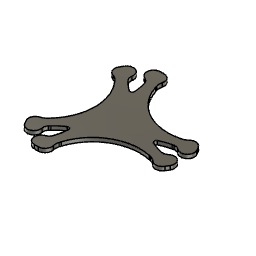
slot_solve (Autodesk Fusion 360 design; units mm, degrees)
Autodesk Fusion 360 part; units mm, degrees
sketch "Sketch1" plane through (0, 0, 0) normal (0, 0, 1) x (1, 0, 0)
  line L0 (0, 0) -> (24.4074, 5.411) construction
  line L1 (1.75, 0) -> (22.5, 0) construction
  dimension "d1" = 25
  dimension "d2" = 12.5
  constraint coincident L0.start origin
  measures "d1" distance of L0.start L0.end
  measures "d2" angle of L0 L1
ref_plane "WorkPlane1" through (0, 0, 20) normal (0, 0, 1) x (1, 0, 0)
sketch "Sketch2" plane through (0, 0, 20) normal (0, 0, 1) x (1, 0, 0)
  line L0 (0, 0) -> (16.8898, 18.4319) construction
  line L1 (1.75, 0) -> (22.5, 0) construction
  dimension "d4" = 25
  dimension "d5" = 47.5
  constraint coincident L0.start origin
  measures "d4" distance of L0.start L0.end
  measures "d5" angle of L0 L1
sketch "Sketch3" plane through (0, 0, 0) normal (0, 0, 1) x (1, 0, 0)
  line L0 (24.4074, 5.411, 0) -> (16.8898, 18.4319, 20) construction
  point P0 (24.4074, 5.411)
  point P1 (16.8898, 18.4319)
ref_plane "WorkPlane2" through (24.4074, 5.411, 0) normal (-0.300451, 0.520397, 0.799322) x (-0.866025, -0.5, 0)
sketch "Sketch4" plane through (24.4074, 5.411, 0) normal (-0.300451, 0.520397, 0.799322) x (-0.866025, -0.5, 0)
  circle A0 centre (0, 0) radius 0.9
  dimension "d7" = 1.8
  constraint coincident A0.centre origin
  measures "d7" diameter of A0
extrude "Extrude1" add sketch "Sketch4" along normal mid plane 20 makes body 1
ref_plane "WorkPlane3" through (0, 0, -1.6) normal (0, 0, 1) x (1, 0, 0)
sketch "Sketch6" plane through (0, 0, -1.6) normal (0, 0, 1) x (1, 0, 0)
  ellipse E0 centre (25.0088, 4.3693) end of major axis (25.5718, 3.3942) minor radius 0.9
sketch "Sketch5" plane through (0, 0, 0) normal (0, 0, 1) x (1, 0, 0)
  ellipse E0 centre (24.4074, 5.411) end of major axis (24.9704, 4.4359) minor radius 0.9
  line L0 (23.515, 5.1567) -> (24.3424, 3.7236) construction
  arc A0 (24.3424, 3.7236) -> (25.9012, 4.6236) centre (25.1218, 4.1736) ccw construction
  line L1 (25.9012, 4.6236) -> (25.0738, 6.0567) construction
  arc A1 (25.0738, 6.0567) -> (23.515, 5.1567) centre (24.2944, 5.6067) ccw construction
  line L2 (24.2944, 5.6067) -> (25.1218, 4.1736) construction
  ellipse E1 centre (25.0088, 4.3693) end of major axis (25.5718, 3.3942) minor radius 0.9
  line L3 (0, 0) -> (24.4074, 5.411) construction
  line L4 (24.7081, 4.8902) -> (0, 0) construction
  line L5 (24.4074, 5.411) -> (24.5179, 4.8525) construction
  line L6 (14.0336, 5.0778) -> (14.8647, 1.3288) construction
  line L7 (14.8647, 1.3288) -> (22.6751, 3.0603) construction
  line L8 (22.6751, 3.0603) -> (21.844, 6.8093) construction
  line L9 (21.844, 6.8093) -> (14.0336, 5.0778) construction
  line L10 (20.3215, 2.4566) -> (21.0327, 2.6143)
  arc A2 (23.1558, 2.0418) -> (27.6333, 5.6236) centre (25.1218, 4.1736) ccw
  line L11 (27.6333, 5.6236) -> (26.8059, 7.0567)
  line L12 (22.6103, 2.7236) -> (22.6103, 2.7236)
  line L13 (20.167, 6.5195) -> (19.4558, 6.3618)
  arc A3 (20.167, 6.5195) -> (22.2452, 7.6587) centre (19.2493, 10.6588) ccw
  arc A4 (23.1558, 2.0418) -> (21.0327, 2.6143) centre (21.5465, 0.2968) ccw
  arc A5 (26.8059, 7.0567) -> (22.2452, 7.6587) centre (24.2944, 5.6067) ccw
  circle A6 centre (15.612, 5.4892) radius 0.4 construction
  line L14 (1.75, 0) -> (22.5, 0)
  line L15 (20.3215, -2.4566) -> (21.0327, -2.6143)
  arc A7 (21.0327, -2.6143) -> (23.1558, -2.0418) centre (21.5465, -0.2968) ccw
  arc A8 (27.6333, -5.6236) -> (23.1558, -2.0418) centre (25.1218, -4.1736) ccw
  line L16 (27.6333, -5.6236) -> (26.8059, -7.0567)
  arc A9 (22.2452, -7.6587) -> (26.8059, -7.0567) centre (24.2944, -5.6067) ccw
  arc A10 (22.2452, -7.6587) -> (20.167, -6.5195) centre (19.2493, -10.6588) ccw
  line L17 (20.167, -6.5195) -> (19.4558, -6.3618)
  arc A11 (-4.2184, 20.0301) -> (19.4558, 6.3618) centre (15.0768, 26.1138) ccw
  arc A12 (20.3215, 2.4566) -> (15.6882, 0.818) centre (24.7004, -17.2954) ccw
  arc A13 (15.6882, 0.818) -> (15.6882, -0.818) centre (16.0952, 0) ccw
  arc A14 (15.6882, -0.818) -> (20.3215, -2.4566) centre (24.7004, 17.2954) ccw
  line L18 (-4.4375, 20.7248) -> (-4.2184, 20.0301)
  arc A15 (-4.49, 23.0943) -> (-4.4375, 20.7248) centre (-0.3938, 21.9998) ccw
  arc A16 (-4.49, 23.0943) -> (-7.2917, 26.7429) centre (-7.2917, 23.8429) ccw
  line L19 (-8.9464, 26.7429) -> (-7.2917, 26.7429)
  arc A17 (-8.9464, 26.7429) -> (-9.8096, 21.0744) centre (-8.9464, 23.8429) ccw
  arc A18 (-8.2523, 19.522) -> (-9.8096, 21.0744) centre (-10.5162, 18.8082) ccw
  line L20 (-8.0333, 18.8273) -> (-8.2523, 19.522)
  arc A19 (-7.1357, 13.9954) -> (-8.0333, 18.8273) centre (-27.3285, 12.7435) ccw
  arc A20 (-8.5526, 13.1774) -> (-7.1357, 13.9954) centre (-8.0476, 13.9389) ccw
  arc A21 (-12.2882, 16.3706) -> (-8.5526, 13.1774) centre (2.6281, 30.0389) ccw
  line L21 (-12.2882, 16.3706) -> (-12.7804, 16.9077)
  arc A22 (-13.3461, 19.0326) -> (-12.7804, 16.9077) centre (-11.0303, 18.5114) ccw
  arc A23 (-13.3461, 19.0326) -> (-18.6868, 21.1193) centre (-16.1754, 19.6693) ccw
  line L22 (-18.6868, 21.1193) -> (-19.5142, 19.6863)
  arc A24 (-19.5142, 19.6863) -> (-17.7553, 15.4356) centre (-17.0027, 18.2363) ccw
  arc A25 (-15.7295, 14.2054) -> (-17.7553, 15.4356) centre (-18.8555, 11.341) ccw
  line L23 (-15.7295, 14.2054) -> (-15.2374, 13.6683)
  arc A26 (-15.2374, -13.6683) -> (-15.2374, 13.6683) centre (-30.1537, 0) ccw
  line L24 (-15.7295, -14.2054) -> (-15.2374, -13.6683)
  arc A27 (-17.7553, -15.4356) -> (-15.7295, -14.2054) centre (-18.8555, -11.341) ccw
  arc A28 (-17.7553, -15.4356) -> (-19.5142, -19.6863) centre (-17.0027, -18.2363) ccw
  line L25 (-18.6868, -21.1193) -> (-19.5142, -19.6863)
  arc A29 (-18.6868, -21.1193) -> (-13.3461, -19.0326) centre (-16.1754, -19.6693) ccw
  arc A30 (-12.7804, -16.9077) -> (-13.3461, -19.0326) centre (-11.0303, -18.5114) ccw
  line L26 (-12.2882, -16.3706) -> (-12.7804, -16.9077)
  arc A31 (-8.5526, -13.1774) -> (-12.2882, -16.3706) centre (2.6281, -30.0389) ccw
  arc A32 (-7.1357, -13.9954) -> (-8.5526, -13.1774) centre (-8.0476, -13.9389) ccw
  arc A33 (-8.0333, -18.8273) -> (-7.1357, -13.9954) centre (-27.3285, -12.7435) ccw
  line L27 (-8.0333, -18.8273) -> (-8.2523, -19.522)
  arc A34 (-9.8096, -21.0744) -> (-8.2523, -19.522) centre (-10.5162, -18.8082) ccw
  arc A35 (-9.8096, -21.0744) -> (-8.9464, -26.7429) centre (-8.9464, -23.8429) ccw
  line L28 (-8.9464, -26.7429) -> (-7.2917, -26.7429)
  arc A36 (-7.2917, -26.7429) -> (-4.49, -23.0943) centre (-7.2917, -23.8429) ccw
  arc A37 (-4.4375, -20.7248) -> (-4.49, -23.0943) centre (-0.3938, -21.9998) ccw
  line L29 (-4.4375, -20.7248) -> (-4.2184, -20.0301)
  arc A38 (19.4558, -6.3618) -> (-4.2184, -20.0301) centre (15.0768, -26.1138) ccw
  point P0 (24.7081, 4.8902)
  point P1 (14.4492, 3.2033)
  dimension "d11" = 107.5
  dimension "d12" = 0.1939
  dimension "d13" = 0.5693
  dimension "d14" = 3.84
  dimension "d15" = 8
  dimension "d16" = 14.8
  dimension "d17" = 2
  dimension "d19" = 1.7
  dimension "d21" = 1.7
  dimension "d22" = 2
  dimension "d23" = 2
  dimension "d24" = 1.63
  dimension "d25" = 0.06
  dimension "d26" = 0.8
  dimension "d38" = 360
  constraint tangent L0 A0
  constraint tangent A0 L1
  constraint parallel L0 L1
  constraint tangent L1 A1
  constraint tangent L0 A1
  constraint tangent E0 L1
  constraint tangent L1 E1
  constraint tangent E0 L0
  constraint tangent E0 A1
  constraint tangent A0 E1
  constraint coincident L2 P0
  constraint midpoint L2 P0
  constraint coincident P0 L4.start
  constraint coincident L3.start L4.end
  constraint coincident E0.centre L3.end
  constraint coincident L4 L5.end
  constraint perpendicular L4 L5
  constraint perpendicular L6 L7
  constraint parallel L6 L8
  constraint parallel L7 L9
  constraint parallel L3 L9
  constraint midpoint L6 P1
  constraint coincident L3 P1
  constraint parallel L7 L10
  constraint parallel L9 L13
  constraint tangent L13 A3
  constraint tangent A3 A5
  constraint tangent L10 A4
  constraint tangent A2 A4
  constraint concentric A0 A2
  constraint parallel L1 L11
  constraint concentric A1 A5
  constraint parallel L0 L12
  constraint tangent L11 A5
  constraint tangent A2 L11
  constraint symmetric L10.start L14 L15.start
  constraint symmetric L10.end L14 L15.end
  constraint symmetric A2.end L14 A8.start
  constraint symmetric A2 L14 A8
  constraint symmetric L11.end L14 L16.end
  constraint symmetric L13.start L14 A10.end
  constraint symmetric L13.end L14 L17.end
  constraint symmetric A3.end L14 A9.start
  constraint symmetric A3 L14 A10
  constraint symmetric A2.start L14 A7.end
  constraint symmetric A4 L14 A7
  constraint symmetric A5 L14 A9
  constraint tangent L13 A11
  constraint tangent A6 A11
  constraint equal L10 L13
  constraint tangent L10 A12
  constraint equal A11 A12
  constraint tangent A12 A13
  constraint symmetric L14 A12.end A13.end
  constraint symmetric L14 A12 A14
  constraint coincident A13.end A14.start
  constraint coincident A11.start L18.end
  constraint tangent L6 A13
  measures "d11" angle of L0 L3
  measures "d12" distance of P0 L5
  measures "d13" distance of E0.centre L5.end
  measures "d14" distance of L6.start L6.end
  measures "d15" distance of L6.start L8.end
  measures "d16" distance of L3.start L6
  measures "d17" distance of L3 L10
  measures "d19" distance of L8 L10.end
  measures "d21" distance of L8 L13.start
  measures "d22" distance of L3 L13
  measures "d23" distance of A1 A5
  measures "d24" distance of L6 A6.centre
  measures "d25" distance of L9 A6.centre
  measures "d26" diameter of A6
extrude "Extrude2" add sketch "Sketch5" against normal up to surface (1.6 mm away) separate body contours E0 E1 | E0 E1 | E0 E1 | L10 A2 L11 L13 A3 A4 A5 L15 A7 A8 L16 A9 A10 L17 A11 A12 A13 A14 L18 A15 A16 L19 A17 A18 L20 A19 A20 A21 L21 A22 A23 L22 A24 A25 L23 A26 L24 A27 A28 L25 A29 A30 L26 A31 A32 A33 L27 A34 A35 L28 A36 A37 L29 A38 makes body 2
sketch "Sketch7" plane through (0, 0, 0) normal (0, 0, 1) x (1, 0, 0)
  line L0 (19.4558, -6.3618) -> (20.167, -6.5195)
  arc A0 (22.2452, -7.6587) -> (20.167, -6.5195) centre (19.2493, -10.6588) ccw
  arc A1 (22.2452, -7.6587) -> (26.8059, -7.0567) centre (24.2944, -5.6067) ccw
  line L1 (26.8059, -7.0567) -> (27.6333, -5.6236)
  arc A2 (27.6333, -5.6236) -> (23.1558, -2.0418) centre (25.1218, -4.1736) ccw
  arc A3 (21.0327, -2.6143) -> (23.1558, -2.0418) centre (21.5465, -0.2968) ccw
  line L2 (21.0327, -2.6143) -> (20.3215, -2.4566)
  line L3 (20.3215, 2.4566) -> (21.0327, 2.6143)
  arc A4 (23.1558, 2.0418) -> (21.0327, 2.6143) centre (21.5465, 0.2968) ccw
  arc A5 (23.1558, 2.0418) -> (27.6333, 5.6236) centre (25.1218, 4.1736) ccw
  line L4 (27.6333, 5.6236) -> (26.8059, 7.0567)
  arc A6 (26.8059, 7.0567) -> (22.2452, 7.6587) centre (24.2944, 5.6067) ccw
  arc A7 (20.167, 6.5195) -> (22.2452, 7.6587) centre (19.2493, 10.6588) ccw
  line L5 (20.167, 6.5195) -> (19.4558, 6.3618)
  arc A8 (-4.2184, 20.0301) -> (19.4558, 6.3618) centre (15.0768, 26.1138) ccw
  arc A9 (15.6882, -0.818) -> (20.3215, -2.4566) centre (24.7004, 17.2954) ccw
  arc A10 (15.6882, 0.818) -> (15.6882, -0.818) centre (16.0952, 0) ccw
  arc A11 (20.3215, 2.4566) -> (15.6882, 0.818) centre (24.7004, -17.2954) ccw
  line L6 (-4.2184, 20.0301) -> (-4.4375, 20.7248)
  arc A12 (-4.49, 23.0943) -> (-4.4375, 20.7248) centre (-0.3938, 21.9998) ccw
  arc A13 (-4.49, 23.0943) -> (-7.2917, 26.7429) centre (-7.2917, 23.8429) ccw
  line L7 (-7.2917, 26.7429) -> (-8.9464, 26.7429)
  arc A14 (-8.9464, 26.7429) -> (-9.8096, 21.0744) centre (-8.9464, 23.8429) ccw
  arc A15 (-8.2523, 19.522) -> (-9.8096, 21.0744) centre (-10.5162, 18.8082) ccw
  line L8 (-8.2523, 19.522) -> (-8.0333, 18.8273)
  arc A16 (-7.1357, 13.9954) -> (-8.0333, 18.8273) centre (-27.3285, 12.7435) ccw
  arc A17 (-8.5526, 13.1774) -> (-7.1357, 13.9954) centre (-8.0476, 13.9389) ccw
  arc A18 (-12.2882, 16.3706) -> (-8.5526, 13.1774) centre (2.6281, 30.0389) ccw
  line L9 (-12.2882, 16.3706) -> (-12.7804, 16.9077)
  arc A19 (-13.3461, 19.0326) -> (-12.7804, 16.9077) centre (-11.0303, 18.5114) ccw
  arc A20 (-13.3461, 19.0326) -> (-18.6868, 21.1193) centre (-16.1754, 19.6693) ccw
  line L10 (-18.6868, 21.1193) -> (-19.5142, 19.6863)
  arc A21 (-19.5142, 19.6863) -> (-17.7553, 15.4356) centre (-17.0027, 18.2363) ccw
  arc A22 (-15.7295, 14.2054) -> (-17.7553, 15.4356) centre (-18.8555, 11.341) ccw
  line L11 (-15.7295, 14.2054) -> (-15.2374, 13.6683)
  arc A23 (-15.2374, -13.6683) -> (-15.2374, 13.6683) centre (-30.1537, 0) ccw
  line L12 (-15.2374, -13.6683) -> (-15.7295, -14.2054)
  arc A24 (-17.7553, -15.4356) -> (-15.7295, -14.2054) centre (-18.8555, -11.341) ccw
  arc A25 (-17.7553, -15.4356) -> (-19.5142, -19.6863) centre (-17.0027, -18.2363) ccw
  line L13 (-19.5142, -19.6863) -> (-18.6868, -21.1193)
  arc A26 (-18.6868, -21.1193) -> (-13.3461, -19.0326) centre (-16.1754, -19.6693) ccw
  arc A27 (-12.7804, -16.9077) -> (-13.3461, -19.0326) centre (-11.0303, -18.5114) ccw
  line L14 (-12.7804, -16.9077) -> (-12.2882, -16.3706)
  arc A28 (-8.5526, -13.1774) -> (-12.2882, -16.3706) centre (2.6281, -30.0389) ccw
  arc A29 (-7.1357, -13.9954) -> (-8.5526, -13.1774) centre (-8.0476, -13.9389) ccw
  arc A30 (-8.0333, -18.8273) -> (-7.1357, -13.9954) centre (-27.3285, -12.7435) ccw
  line L15 (-8.0333, -18.8273) -> (-8.2523, -19.522)
  arc A31 (-9.8096, -21.0744) -> (-8.2523, -19.522) centre (-10.5162, -18.8082) ccw
  arc A32 (-9.8096, -21.0744) -> (-8.9464, -26.7429) centre (-8.9464, -23.8429) ccw
  line L16 (-8.9464, -26.7429) -> (-7.2917, -26.7429)
  arc A33 (-7.2917, -26.7429) -> (-4.49, -23.0943) centre (-7.2917, -23.8429) ccw
  arc A34 (-4.4375, -20.7248) -> (-4.49, -23.0943) centre (-0.3938, -21.9998) ccw
  line L17 (-4.4375, -20.7248) -> (-4.2184, -20.0301)
  arc A35 (19.4558, -6.3618) -> (-4.2184, -20.0301) centre (15.0768, -26.1138) ccw
hidden bodies 1
equation "d5 = 60 deg - 12.5 deg"
